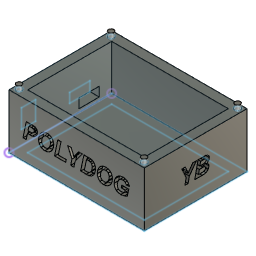
Boitier Arduino v1 (Autodesk Fusion 360 design; units mm, degrees)
Autodesk Fusion 360 part; units mm, degrees
sketch "Esquisse1" plane through (0, 0, 0) normal (0, 0, 1) x (1, 0, 0)
  line L0 (-46.7984, 35.5123) -> (40.2016, 35.5123)
  line L1 (40.2016, 35.5123) -> (40.2016, -30.4877)
  line L2 (40.2016, -30.4877) -> (-46.7984, -30.4877)
  line L3 (-46.7984, -30.4877) -> (-46.7984, 35.5123)
  line L4 (-40.7984, -24.4877) -> (-40.7984, 29.5123)
  line L5 (-40.7984, 29.5123) -> (34.2016, 29.5123)
  line L6 (34.2016, 29.5123) -> (34.2016, -24.4877)
  line L7 (34.2016, -24.4877) -> (-40.7984, -24.4877)
  dimension "d1" = 6
  dimension "d10" = 87
  dimension "d11" = 66
  constraint horizontal L0
  constraint vertical L1
  constraint horizontal L2
  constraint vertical L3
  measures "d10" distance of L1 L3
  measures "d11" distance of L0 L2
extrude "Extrusion1" add sketch "Esquisse1" along normal blind 6 contours L4 L5 L6 L7
extrude "Extrusion2" add sketch "Esquisse1" along normal blind 35
sketch "Esquisse2" plane through (-46.7984, 0, 0) normal (-1, 0, 0) x (0, -1, 0)
  line L0 (-35.5123, 0) -> (30.4877, 0)
  line L1 (30.4877, 0) -> (30.4877, 35)
  line L2 (30.4877, 35) -> (-35.5123, 35)
  line L3 (-35.5123, 35) -> (-35.5123, 0)
  line L4 (-21.5123, 14.024) -> (-8.5123, 14.024)
  line L5 (-8.5123, 14.024) -> (-8.5123, 8)
  line L6 (-8.5123, 8) -> (-21.5123, 8)
  line L7 (-21.5123, 8) -> (-21.5123, 14.024)
  line L8 (13.4517, 21) -> (22.4877, 21)
  line L9 (22.4877, 21) -> (22.4877, 9)
  line L10 (22.4877, 9) -> (13.4517, 9)
  line L11 (13.4517, 9) -> (13.4517, 21)
  line L12 (30.4877, 0) -> (-35.5123, 0)
  constraint horizontal L4
  constraint vertical L5
  constraint horizontal L6
  constraint vertical L7
  constraint horizontal L8
  constraint vertical L9
  constraint horizontal L10
  constraint vertical L11
extrude "Extrusion3" cut sketch "Esquisse2" against normal blind 10 contours L4 L5 L6 L7 | L8 L9 L10 L11
sketch "Esquisse3" plane through (0, 0, 35) normal (0, 0, 1) x (-1, 0, 0)
  line L0 (-34.2016, -29.5123) -> (-34.2016, 24.4877)
  line L1 (-34.2016, 24.4877) -> (40.7984, 24.4877)
  line L2 (40.7984, 24.4877) -> (40.7984, -29.5123)
  line L3 (40.7984, -29.5123) -> (-34.2016, -29.5123)
  line L4 (46.7984, 30.4877) -> (-40.2016, 30.4877)
  line L5 (-40.2016, 30.4877) -> (-40.2016, -35.5123)
  line L6 (-40.2016, -35.5123) -> (46.7984, -35.5123)
  line L7 (46.7984, -35.5123) -> (46.7984, 30.4877)
  circle A0 centre (43.7129, -32.1036) radius 1.75
  circle A1 centre (43.8897, 26.9398) radius 1.75
  circle A2 centre (-37.0739, -32.6339) radius 1.75
  circle A3 centre (-37.0739, 27.4701) radius 1.75
extrude "Extrusion4" add sketch "Esquisse3" along normal blind 3 contours A0 | A1 | A2 | A3
sketch "Esquisse4" plane through (0, -30.4877, 0) normal (0, -1, 0) x (1, 0, 0)
  line L0 (-46.7984, 0) -> (40.2016, 0)
  line L1 (40.2016, 0) -> (40.2016, 35)
  line L2 (40.2016, 35) -> (-46.7984, 35)
  line L3 (-46.7984, 35) -> (-46.7984, 0)
  line L4 (-44.8974, 2.3418) -> (37.6572, 2.3418) construction
  line L5 (37.6572, 2.3418) -> (37.6572, 33.2792) construction
  line L6 (37.6572, 33.2792) -> (-44.8974, 33.2792) construction
  line L7 (-44.8974, 33.2792) -> (-44.8974, 2.3418) construction
  dimension "d33" = 10
  text T0 "POLYDOG" font "Arial" height 10 bold italic align centre middle in box 82.5546 x 30.9374 at (-44.8974, 2.3418) x (1, 0) y (0, 1) spacing 1 kerned
extrude "Extrusion5" cut sketch "Esquisse4" against normal blind 3 text T0
sketch "Esquisse5" plane through (40.2016, 0, 0) normal (1, 0, 0) x (0, 1, 0)
  line L0 (-30.4877, 0) -> (35.5123, 0)
  line L1 (35.5123, 0) -> (35.5123, 35)
  line L2 (35.5123, 35) -> (-30.4877, 35)
  line L3 (-30.4877, 35) -> (-30.4877, 0)
  line L4 (-28.8013, 1.1722) -> (33.7776, 1.1722) construction
  line L5 (33.7776, 1.1722) -> (33.7776, 33.3455) construction
  line L6 (33.7776, 33.3455) -> (-28.8013, 33.3455) construction
  line L7 (-28.8013, 33.3455) -> (-28.8013, 1.1722) construction
  dimension "d36" = 10
  text T0 "YB" font "Arial" height 10 bold italic align centre middle in box 62.5789 x 32.1733 at (-28.8013, 1.1722) x (1, 0) y (0, 1) spacing 1 kerned
extrude "Extrusion6" cut sketch "Esquisse5" against normal blind 3 text T0
equation "d1 = epaisseur"
equation "d2 = epaisseur"
equation "d4 = hauteur"
equation "longueur = 87 mm"
equation "largeur = 66 mm"
equation "hauteur = 35 mm"
equation "epaisseur = 6 mm"
equation "d10 = longueur"
equation "d11 = largeur"
equation "h1 = 6.024 mm"
equation "l1 = 13 mm"
equation "h2 = 12 mm"
equation "l2 = 9.036 mm"
